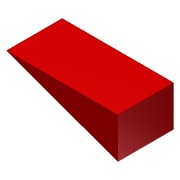
# Autodesk Inventor part: LaunchAngle
Saved by Autodesk Inventor 2012 (Build 160160000, 160)
## iProperties
Created: 2013-01-19
Part Number: LaunchAngle
Material: Default
Document SubType Name: Modeling
Designer: JesseK
Density: 1 g/cm^3
Mass: 11.9288 g
Surface Area: 40.7236 cm^2
Volume: 11.9288 cm^3
Author: JesseK
Autodesk Inventor part; units mm, degrees
ref_plane "YZ Plane" through (0, 0, 0) normal (1, 0, 0) x (0, 1, 0)
ref_plane "XZ Plane" through (0, 0, 0) normal (0, 1, 0) x (-1, 0, 0)
ref_plane "XY Plane" through (0, 0, 0) normal (0, 0, 1) x (1, 0, 0)
sketch "Sketch1" plane through (0, 0, 0) normal (0, 0, 1) x (1, 0, 0)
  line L0 (0, 0) -> (0, 18.4897)
  line L1 (0, 18.4897) -> (-50.8, 18.4897)
  line L2 (-50.8, 18.4897) -> (0, 0)
  dimension "d0" = 20
  dimension "d1" = 50.8
  constraints: 6 end point, 1 horizontal, 1 vertical
  measures "d0" angle of L1 L2
  measures "d1" distance of L0.end L1.end
extrude "Extrusion1" add sketch "Sketch1" along normal blind 25.4
body "Solid1"
